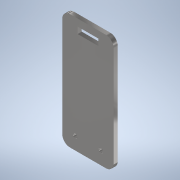
# Autodesk Inventor part: SP40V1 Chapa Base
Saved by Autodesk Inventor 2021.2 (Build 252289000, 289)
## iProperties
Created: 2026-08-24
Part Number: SP40V1 Chapa Base
Material: Generic
Document SubType Name: Sheet Metal
Designer: nelso
Density: 1 g/cm^3
Sheet Metal Rule: Default_mm
Appearance: Stainless - Polished
Author: nelso
Autodesk Inventor part; units mm, degrees
ref_plane "YZ Plane" through (0, 0, 0) normal (1, 0, 0) x (0, 1, 0)
ref_plane "XZ Plane" through (0, 0, 0) normal (0, 1, 0) x (-1, 0, 0)
ref_plane "XY Plane" through (0, 0, 0) normal (0, 0, 1) x (1, 0, 0)
sketch "Sketch1" plane through (0, 0, 0) normal (0, 1, 0) x (-1, 0, 0)
  line L0 (20, 45) -> (-20, 45)
  line L1 (-20, 45) -> (-20, -45)
  line L2 (-20, -45) -> (20, -45)
  line L3 (20, -45) -> (20, 45)
  line L4 (20, 45) -> (-20, -45) construction
  line L5 (-20, 45) -> (20, -45) construction
  point P0 (0, 0)
  dimension "d0" = 40
  dimension "d1" = 90
  measures "d0" distance of L2.end L1.end
  measures "d1" distance of L1.end L0.end
extrude "Plate1" add sketch "Sketch1" along normal blind 3.2
sketch "Sketch2" plane through (0, 3.2, 0) normal (0, 1, 0) x (1, 0, 0)
  line L0 (-20, -45) -> (20, -45) projected
  line L1 (0, -45) -> (0, 35)
  line L2 (0, 35) -> (-10, 35)
  point P0 (0, 0)
  point P1 (10, 35)
  point P2 (10, 35)
  dimension "d3" = 80
  dimension "d4" = 10
  constraints: 4 end point, 2 coincident, 2 symmetric about line, 1 horizontal, 1 midpoint, 1 vertical
  measures "d3" distance of L1.start L1.end
  measures "d4" distance of L1.end L2.end
hole "Hole1" at (-10, 3.2, -35) at (10, 3.2, -35) direction (0, -1, 0) diameter 3.4 depth 3.2 tip angle 118 clearance for "Countersunk Flat Head Screw ISO 2009/7046" size "M3" standard "ISO"
sketch "Sketch4" plane through (0, 0, 0) normal (0, -1, 0) x (1, 0, 0)
  line L0 (8, 39.559) -> (-8, 39.559)
  line L1 (-8, 39.559) -> (-8, 34.559)
  line L2 (-8, 34.559) -> (8, 34.559)
  line L3 (8, 34.559) -> (8, 39.559)
  line L4 (8, 39.559) -> (-8, 34.559) construction
  line L5 (-8, 39.559) -> (8, 34.559) construction
  line L6 (-20, 45) -> (20, 45) projected
  point P0 (0, 0)
  point P1 (0, 37.059)
  dimension "d12" = 16
  dimension "d13" = 5
  dimension "d17" = 7.941
  constraints: 12 end point, 2 midpoint, 2 parallel, 1 horizontal, 1 perpendicular
  measures "d12" distance of L2.end L1.end
  measures "d13" distance of L1.end L0.end
  measures "d17" distance from line of L6 point (0, 37.059)
extrude "Cut1" cut sketch "Sketch4" against normal blind 3.2
fillet "Corner Round1" radius 6 4 edges at (20, 1.6, 45) (-20, 1.6, 45) (20, 1.6, -45) (-20, 1.6, -45)
equation "\"d10\" = Thickness"
equation "\"d14\" = Thickness"
equation "\"d2\" = Thickness"
equation "\"BendReliefWidth\" = Thickness"
equation "\"BendReliefDepth\" = 0.5 * Thickness"
equation "\"CornerReliefSize\" = 4 * Thickness"
equation "\"MinimumRemnant\" = 2 * Thickness"
equation "\"TransitionRadius\" = BendRadius"
equation "\"JacobiRadiusSize\" = BendRadius"
equation "\"GapSize\" = Thickness"
equation "\"Thickness\" = 3.2"
equation "\"BendRadius\" = 1.516"
body "Solid1"
